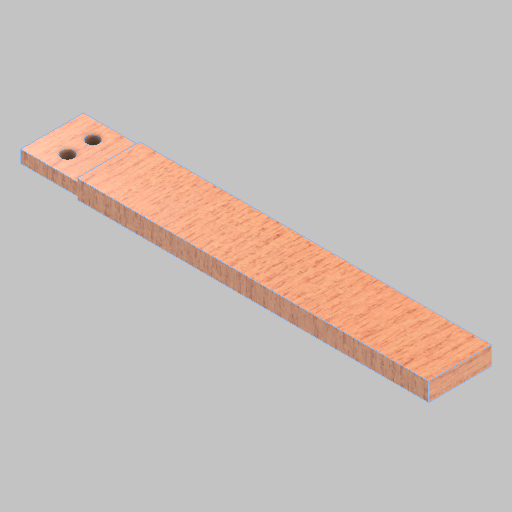
# Autodesk Inventor part: Pás - Hastes
Saved by Autodesk Inventor 2025.2 (Build 292293000, 293)
## iProperties
Created: 2024-04-26
Part Number: Pás - Hastes
Material: Genérico
Document SubType Name: Modeling
Designer: phmca
Density: 1 g/cm^3
Appearance: Acetinada manchada - Azul
Author: phmca
Autodesk Inventor part; units mm, degrees
ref_plane "YZ Plane" through (0, 0, 0) normal (1, 0, 0) x (0, 1, 0)
ref_plane "XZ Plane" through (0, 0, 0) normal (0, 1, 0) x (-1, 0, 0)
ref_plane "XY Plane" through (0, 0, 0) normal (0, 0, 1) x (1, 0, 0)
sketch "Esboço1" plane through (0, 0, 0) normal (0, 0, 1) x (1, 0, 0)
  line L0 (-162.5, -7.5) -> (-117.5, -7.5) construction
  line L1 (162.5, -7.5) -> (162.5, 7.5)
  line L2 (162.5, 7.5) -> (-117.5, 7.5)
  line L3 (-162.5, 7.5) -> (-162.5, 5) construction
  line L4 (-162.5, -7.5) -> (162.5, 7.5) construction
  line L5 (162.5, -7.5) -> (-162.5, 7.5) construction
  line L6 (-162.5, -5) -> (-117.5, -5)
  line L7 (-117.5, 5) -> (-162.5, 5)
  line L8 (-117.5, 5) -> (-117.5, 7.5)
  line L9 (-117.5, -5) -> (-117.5, -7.5)
  line L10 (-117.5, 5) -> (-117.5, -5) construction
  line L11 (-117.5, 0) -> (0, 0) construction
  line L12 (-162.5, 5) -> (-162.5, -5)
  line L13 (-162.5, -5) -> (-162.5, -7.5) construction
  line L14 (-117.5, -7.5) -> (162.5, -7.5)
  line L15 (-117.5, 7.5) -> (-162.5, 7.5) construction
  dimension "d0" = 325
  dimension "d1" = 15
  dimension "d2" = 10
  dimension "d3" = 45
  constraints: 32 end point, 8 parallel, 4 horizontal, 4 perpendicular, 3 midpoint, 2 vertical, 1 point on line
  measures "d0" distance of L3.start L1.end
  measures "d1" distance of L1.end L1.start
  measures "d2" distance between parallel lines of L6 L7
  measures "d3" distance between parallel lines of L8 L12
extrude "Extrusão1" add sketch "Esboço1" along normal mid plane 50
sketch "Esboço2" plane through (-162.5, 5, 25) normal (0, 1, 0) x (1, 0, 0)
  line L0 (0, 0) -> (0, 50) projected
  line L1 (45, 50) -> (45, 0) projected
  circle A0 centre (22.5, 35) radius 5
  circle A1 centre (22.5, 15) radius 5
  line L2 (22.5, 15) -> (22.5, 35)
  line L3 (0, 50) -> (45, 50) projected
  line L4 (22.5, 50) -> (22.5, 74.6859)
  line L5 (22.5, 25) -> (-20.9828, 25) construction
  line L6 (0, 25) -> (-37.1648, 25) construction
  point P0 (162.5, 25)
  dimension "d14" = 10
  dimension "d15" = 10
  dimension "d16" = 20
  constraints: 8 end point, 3 midpoint, 2 centre point, 2 collinear, 2 horizontal, 2 vertical
  measures "d14" diameter of A0
  measures "d15" diameter of A1
  measures "d16" distance of L2.start L2.end
extrude "Extrusão2" cut sketch "Esboço2" against normal up to surface (10 mm away)
sketch "ref. Motor" plane through (-117.5, -7.5, 25) normal (0, -1, 0) x (1, 0, 0)
  line L0 (280, -50) -> (280, 0) projected
  line L1 (280, -25) -> (270, -25) construction
  line L2 (270, -25) -> (270, 54.6764) construction
  point P0 (117.5, -25)
  dimension "d13" = 10
  constraints: 4 end point, 1 horizontal, 1 midpoint, 1 vertical
  measures "d13" distance of L1.start L1.end
equation "\"d15\" = d14"
